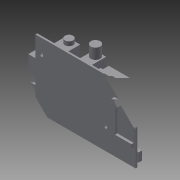
# Autodesk Inventor part: PCB
Saved by Autodesk Inventor 2014 (Build 180170000, 170)
## iProperties
Created: 2013-05-24
Part Number: PCB
Material: Generisch
Document SubType Name: Modeling
Designer: hartmann
Density: 1 g/cm^3
Appearance: Vorgabe
Author: hartmann
Autodesk Inventor part; units mm, degrees
ref_plane "YZ Plane" through (0, 0, 0) normal (1, 0, 0) x (0, 1, 0)
ref_plane "XZ Plane" through (0, 0, 0) normal (0, 1, 0) x (-1, 0, 0)
ref_plane "XY Plane" through (0, 0, 0) normal (0, 0, 1) x (1, 0, 0)
sketch "Skizze1" plane through (0, 0, 0) normal (0, 1, 0) x (-1, 0, 0)
  line L0 (0, 0) -> (85, 0)
  line L1 (85, 0) -> (85, 56)
  line L2 (85, 56) -> (0, 56)
  line L3 (0, 56) -> (0, 0)
  dimension "d0" = 85
  dimension "d1" = 56
  constraints: 8 end point, 2 parallel, 1 horizontal, 1 perpendicular
  measures "d0" distance of L1.end L2.end
  measures "d1" distance of L0.end L1.end
extrude "Extrusion1" add sketch "Skizze1" along normal blind 1.5
sketch "Skizze2" plane through (0, 1.5, 0) normal (0, 1, 0) x (1, 0, 0)
  line L0 (0, 0) -> (-85, 0) projected
  line L1 (-93.3944, -17.2) -> (-72.3944, -17.2)
  line L2 (-72.3944, -17.2) -> (-72.3944, -1.2)
  line L3 (-72.3944, -1.2) -> (-93.3944, -1.2)
  line L4 (-93.3944, -1.2) -> (-93.3944, -17.2)
  dimension "d4" = 21
  dimension "d5" = 16
  dimension "d6" = 1.2
  constraints: 8 end point, 2 parallel, 1 horizontal, 1 perpendicular
  measures "d4" distance of L2.end L3.end
  measures "d5" distance of L3.end L1.start
  measures "d6" distance between parallel lines of L0 L3
extrude "Extrusion2" add sketch "Skizze2" along normal blind 13.4
sketch "Skizze3" plane through (0, 1.5, 0) normal (0, 1, 0) x (1, 0, 0)
  line L0 (-72.3944, -17.2) -> (-85, -17.2) projected
  line L1 (-85, -17.2) -> (-85, -56) projected
  line L2 (-92.5, -23.8) -> (-75.1, -23.8)
  line L3 (-75.1, -23.8) -> (-75.1, -37)
  line L4 (-75.1, -37) -> (-92.5, -37)
  line L5 (-92.5, -37) -> (-92.5, -23.8)
  dimension "d9" = 7.5
  dimension "d10" = 17.4
  dimension "d11" = 13.2
  dimension "d12" = 6.6
  constraints: 8 end point, 2 parallel, 1 horizontal, 1 perpendicular
  measures "d9" distance between parallel lines of L1 L5
  measures "d10" distance of L2.start L2.end
  measures "d11" distance of L2.end L3.end
  measures "d12" distance between parallel lines of L0 L2
extrude "Extrusion3" add sketch "Skizze3" along normal blind 16
sketch "Skizze4" plane through (0, 1.5, 0) normal (0, 1, 0) x (1, 0, 0)
  line L0 (0, 0) -> (-85, 0) projected
  line L1 (-72.3944, -1.2) -> (-72.3944, -17.2) projected
  line L2 (-57.3944, 1) -> (-42.3944, 1)
  line L3 (-42.3944, 1) -> (-42.3944, -10.8)
  line L4 (-42.3944, -10.8) -> (-57.3944, -10.8)
  line L5 (-57.3944, -10.8) -> (-57.3944, 1)
  dimension "d15" = 1
  dimension "d16" = 15
  dimension "d17" = 11.8
  dimension "d18" = 15
  constraints: 8 end point, 2 parallel, 1 horizontal, 1 perpendicular
  measures "d15" distance between parallel lines of L0 L2
  measures "d16" distance of L3.end L4.end
  measures "d17" distance of L2.end L3.end
  measures "d18" distance between parallel lines of L5 L1
extrude "Extrusion4" add sketch "Skizze4" along normal blind 5.5
sketch "Skizze5" plane through (0, 1.5, 0) normal (0, 1, 0) x (1, 0, 0)
  line L0 (-85, -37) -> (-85, -56) projected
  line L1 (-85, -56) -> (0, -56) projected
  line L2 (-58.5, -44.5) -> (-70.5, -44.5)
  line L3 (-70.5, -44.5) -> (-70.5, -56)
  line L4 (-70.5, -56) -> (-58.5, -56)
  line L5 (-58.5, -56) -> (-58.5, -44.5)
  line L6 (-70.5, -56) -> (-58.5, -56)
  dimension "d21" = 11.5
  dimension "d22" = 12
  dimension "d23" = 14.5
  constraints: 10 end point, 2 parallel, 1 collinear, 1 horizontal, 1 perpendicular, 1 point on line
  measures "d21" distance of L4.end L2.start
  measures "d22" distance of L2.start L2.end
  measures "d23" distance between parallel lines of L0 L3
extrude "Extrusion5" add sketch "Skizze5" along normal blind 10
sketch "Skizze6" plane through (-85, 0, 56) normal (0, 0, 1) x (1, 0, 0)
  line L0 (14.5, 11.5) -> (26.5, 11.5) projected
  circle A0 centre (20.5, 8) radius 3.5
  dimension "d26" = 7
  dimension "d27" = 3.5
  constraints: 1 centre point
  measures "d26" diameter of A0
  measures "d27" distance from line of L0 A0.centre
extrude "Extrusion6" add sketch "Skizze6" along normal blind 3.5
sketch "Skizze7" plane through (0, 1.5, 0) normal (0, 1, 0) x (1, 0, 0)
  line L0 (-58.5, -44.5) -> (-58.5, -56) projected
  line L1 (-58.5, -56) -> (0, -56) projected
  line L2 (-51, -43.5) -> (-41, -43.5)
  line L3 (-41, -43.5) -> (-41, -53.5)
  line L4 (-41, -53.5) -> (-51, -53.5)
  line L5 (-51, -53.5) -> (-51, -43.5)
  dimension "d30" = 10
  dimension "d31" = 10
  dimension "d32" = 2.5
  dimension "d33" = 7.5
  constraints: 8 end point, 2 parallel, 1 horizontal, 1 perpendicular
  measures "d30" distance of L2.start L2.end
  measures "d31" distance of L2.end L3.end
  measures "d32" distance between parallel lines of L4 L1
  measures "d33" distance between parallel lines of L5 L0
extrude "Extrusion7" add sketch "Skizze7" along normal blind 14.5
sketch "Skizze8" plane through (-51, 1.5, 53.5) normal (0, 0, 1) x (1, 0, 0)
  line L0 (0, 14.5) -> (10, 14.5) projected
  circle A0 centre (5, 10.5) radius 4
  point P0 (51, -1.5)
  dimension "d36" = 8
  dimension "d37" = 0
  constraints: 1 centre point
  measures "d36" diameter of A0
  measures "d37" distance edge to line of A0 L0
extrude "Extrusion8" add sketch "Skizze8" along normal blind 9
sketch "Skizze9" plane through (0, 1.5, 0) normal (0, 1, 0) x (1, 0, 0)
  line L0 (-58.5, -56) -> (0, -56) projected
  line L1 (0, -56) -> (0, 0) projected
  line L2 (-1, -55) -> (-33.7, -55)
  line L3 (-33.7, -55) -> (-33.7, -50)
  line L4 (-33.7, -50) -> (-1, -50)
  line L5 (-1, -50) -> (-1, -55)
  dimension "d40" = 32.7
  dimension "d41" = 5
  dimension "d42" = 1
  dimension "d43" = 1
  constraints: 8 end point, 2 parallel, 1 horizontal, 1 perpendicular
  measures "d40" distance of L3.end L4.end
  measures "d41" distance of L4.end L2.start
  measures "d42" distance between parallel lines of L2 L0
  measures "d43" distance between parallel lines of L1 L5
extrude "Extrusion9" add sketch "Skizze9" along normal blind 2.5
sketch "Skizze10" plane through (0, 4, 0) normal (0, 1, 0) x (1, 0, 0)
  line L0 (-33.7, -55) -> (-1, -55) projected
  line L1 (-1, -55) -> (-1, -50) projected
  line L2 (-1, -50) -> (-33.7, -50) projected
  line L3 (-33.7, -50) -> (-33.7, -55) projected
  line L4 (-32.7, -51) -> (-2, -51)
  line L5 (-2, -51) -> (-2, -54)
  line L6 (-2, -54) -> (-32.7, -54)
  line L7 (-32.7, -54) -> (-32.7, -51)
  point P0 (0, 0)
  dimension "d50" = 1
  dimension "d51" = 1
  dimension "d52" = 1
  dimension "d53" = 1
  constraints: 8 end point, 2 parallel, 1 horizontal, 1 perpendicular
  measures "d50" distance between parallel lines of L2 L4
  measures "d51" distance between parallel lines of L1 L5
  measures "d52" distance between parallel lines of L3 L7
  measures "d53" distance between parallel lines of L6 L0
extrude "Extrusion10" add sketch "Skizze10" along normal blind 6 contours L4 L5 L6 L7
sketch "Skizze11" plane through (0, 1.5, 0) normal (0, 1, 0) x (1, 0, 0)
  line L0 (0, -56) -> (0, 0) projected
  line L1 (0, 0) -> (-42.3944, 0) projected
  line L2 (1, -4) -> (-4.6, -4)
  line L3 (-4.6, -4) -> (-4.6, -11.5)
  line L4 (-4.6, -11.5) -> (1, -11.5)
  line L5 (1, -11.5) -> (1, -4)
  dimension "d56" = 1
  dimension "d57" = 7.5
  dimension "d58" = 5.6
  dimension "d59" = 4
  constraints: 8 end point, 2 parallel, 1 horizontal, 1 perpendicular
  measures "d56" distance between parallel lines of L0 L5
  measures "d57" distance between parallel lines of L2 L4
  measures "d58" distance of L3.end L4.end
  measures "d59" distance between parallel lines of L1 L2
extrude "Extrusion11" add sketch "Skizze11" along normal blind 3
sketch "Skizze12" plane through (0, 0, 0) normal (0, -1, 0) x (1, 0, 0)
  line L0 (0, 0) -> (-85, 0) projected
  line L1 (0, 56) -> (0, 0) projected
  line L2 (-1, 43.5) -> (-18, 43.5)
  line L3 (-18, 43.5) -> (-18, 15.5)
  line L4 (-18, 15.5) -> (-1, 15.5)
  line L5 (-1, 15.5) -> (-1, 43.5)
  dimension "d62" = 15.5
  dimension "d63" = 17
  dimension "d64" = 28
  dimension "d65" = 1
  constraints: 8 end point, 2 parallel, 1 horizontal, 1 perpendicular
  measures "d62" distance between parallel lines of L4 L0
  measures "d63" distance of L3.end L4.end
  measures "d64" distance of L2.end L3.end
  measures "d65" distance between parallel lines of L5 L1
extrude "Extrusion12" add sketch "Skizze12" along normal blind 0.5
sketch "Skizze13" plane through (0, -0.5, 0) normal (0, -1, 0) x (1, 0, 0)
  line L0 (-1, 43.5) -> (-18, 43.5) projected
  line L1 (-18, 43.5) -> (-18, 15.5) projected
  line L2 (-18, 15.5) -> (-1, 15.5) projected
  line L3 (-1, 15.5) -> (-1, 43.5) projected
  line L4 (-15, 42.5) -> (-1, 42.5)
  line L5 (-1, 42.5) -> (-1, 18.5)
  line L6 (-1, 18.5) -> (-15, 18.5)
  line L7 (-15, 18.5) -> (-15, 42.5)
  line L8 (-15, 37.5) -> (-10, 42.5)
  line L9 (-15, 37.5) -> (-7.9289, 37.5) construction
  point P0 (0, 0)
  dimension "d69" = 24
  dimension "d70" = 3
  dimension "d71" = 3
  dimension "d72" = 45
  dimension "d73" = 19
  constraints: 12 end point, 3 point on line, 2 horizontal, 2 parallel, 1 equal length, 1 perpendicular
  measures "d69" distance of L6.end L4.start
  measures "d70" distance between parallel lines of L2 L6
  measures "d71" distance between parallel lines of L7 L1
  measures "d72" angle of L9 L8
  measures "d73" distance of L8.start L6.end
extrude "Extrusion13" add sketch "Skizze13" along normal blind 2 contours L3 L4 L7 L6 L2 L1 L0 | L8 L7 L4
sketch "Skizze14" plane through (0, 1.5, 0) normal (0, 1, 0) x (1, 0, 0)
  line L0 (0, 0) -> (-42.3944, 0) projected
  line L1 (-85, -37) -> (-85, -56) projected
  line L2 (-85, -56) -> (-70.5, -56) projected
  line L3 (0, -56) -> (0, -11.5) projected
  circle A0 centre (-25.5, -18) radius 1.45
  circle A1 centre (-80, -43.5) radius 1.45
  dimension "d76" = 2.9
  dimension "d77" = 25.5
  dimension "d78" = 18
  dimension "d79" = 2.9
  dimension "d80" = 5
  dimension "d81" = 12.5
  constraints: 2 centre point
  measures "d76" diameter of A0
  measures "d77" distance from line of L3 A0.centre
  measures "d78" distance from line of L0 A0.centre
  measures "d79" diameter of A1
  measures "d80" distance from line of L1 A1.centre
  measures "d81" distance from line of L2 A1.centre
extrude "Extrusion14" cut sketch "Skizze14" against normal through all
